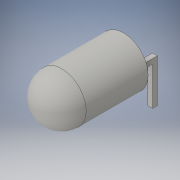
# Autodesk Inventor part: LED
Saved by Autodesk Inventor 2016 (Build 200138000, 138)
## iProperties
Created: 2017-05-28
Part Number: LED
Material: 一般
Document SubType Name: Modeling
Designer: kota
Density: 1 g/cm^3
Appearance: 既定
Author: kota
Autodesk Inventor part; units mm, degrees
ref_plane "YZ Plane" through (0, 0, 0) normal (1, 0, 0) x (0, 1, 0)
ref_plane "XZ Plane" through (0, 0, 0) normal (0, 1, 0) x (-1, 0, 0)
ref_plane "XY Plane" through (0, 0, 0) normal (0, 0, 1) x (1, 0, 0)
sketch "スケッチ1" plane through (0, 0, 0) normal (0, 1, 0) x (-1, 0, 0)
  line L0 (4.5, 2.55) -> (-4.5, 2.55) construction
  line L1 (-4.5, 2.55) -> (-4.5, -2.55) construction
  line L2 (-4.5, -2.55) -> (4.5, -2.55) construction
  line L3 (4.5, -2.55) -> (4.5, 2.55) construction
  line L4 (4.5, 2.55) -> (-4.5, -2.55) construction
  line L5 (-4.5, 2.55) -> (4.5, -2.55) construction
  line L6 (5.4458, 0) -> (-6.2593, 0)
  line L7 (4.5, 0) -> (-4.5, 0)
  arc A0 (4.5, 0) -> (1.95, 2.55) centre (1.95, 0) ccw
  line L8 (-4.5, 2.55) -> (-4.5, 0)
  line L9 (1.95, 2.55) -> (-4.5, 2.55)
  point P0 (0, 0)
  dimension "d0" = 9
  dimension "d1" = 5.1
  constraints: 20 end point, 3 midpoint, 2 collinear, 2 horizontal, 2 parallel, 2 point on circle, 2 point on line, 2 tangent, 1 centre point, 1 perpendicular, 2 other
  measures "d0" distance of L2.end L1.end
  measures "d1" distance of L0.end L1.end
revolve "回転1" add sketch "スケッチ1" angle 360 about axis through (-5.4458, 0, 0) along (1, 0, 0)
sketch "スケッチ2" plane through (4.5, 0, 0) normal (1, 0, 0) x (0, 0, -1)
  line L0 (-3.2936, 0) -> (3.5532, 0)
  line L1 (0, -3.9082) -> (0, 3.9846)
  line L2 (-1.52, 0.25) -> (-1.02, 0.25)
  line L3 (-1.02, 0.25) -> (-1.02, -0.25)
  line L4 (-1.02, -0.25) -> (-1.52, -0.25)
  line L5 (-1.52, -0.25) -> (-1.52, 0.25)
  line L6 (-1.52, 0.25) -> (-1.02, -0.25) construction
  line L7 (-1.02, 0.25) -> (-1.52, -0.25) construction
  line L8 (1.52, 0.25) -> (1.02, 0.25)
  line L9 (1.02, 0.25) -> (1.02, -0.25)
  line L10 (1.02, -0.25) -> (1.52, -0.25)
  line L11 (1.52, 0.25) -> (1.02, -0.25) construction
  line L12 (1.02, 0.25) -> (1.52, -0.25) construction
  line L13 (1.52, -0.25) -> (1.52, 0.25)
  point P0 (0, 0)
  point P1 (-1.27, 0)
  point P2 (-1.27, 0)
  point P3 (1.27, 0)
  point P4 (1.27, 0)
  dimension "d9" = 0.5
  dimension "d10" = 0.5
  dimension "d11" = 1.27
  constraints: 28 end point, 6 symmetric about line, 5 midpoint, 3 horizontal, 2 parallel, 1 perpendicular, 1 point on line, 1 vertical, 4 other
  measures "d9" distance of L3.end L4.end
  measures "d10" distance of L2.end L3.end
  measures "d11" distance of point (0, 0) point (-1.27, 0)
extrude "押し出し1" add sketch "スケッチ2" along normal blind 2
sketch "スケッチ3" plane through (4.5, -0.25, 1.02) normal (0, -1, 0) x (1, 0, 0)
  line L0 (1.5, 0) -> (2, 0)
  line L1 (2, 0) -> (2, 0.5)
  line L2 (2, 0.5) -> (1.5, 0.5)
  line L3 (1.5, 0.5) -> (1.5, 0)
  line L4 (1.5, 0) -> (2, 0.5) construction
  line L5 (2, 0) -> (1.5, 0.5) construction
  line L6 (1.5, -2.04) -> (2, -2.04)
  line L7 (2, -2.04) -> (2, -2.54)
  line L8 (2, -2.54) -> (1.5, -2.54)
  line L9 (1.5, -2.54) -> (1.5, -2.04)
  line L10 (1.5, -2.04) -> (2, -2.54) construction
  line L11 (2, -2.04) -> (1.5, -2.54) construction
  point P0 (-4.5, -1.02)
  point P1 (1.75, 0.25)
  point P2 (1.75, -2.29)
  dimension "d14" = 0.5
  dimension "d15" = 0.5
  dimension "d16" = 0.5
  dimension "d17" = 0.5
  constraints: 24 end point, 4 midpoint, 4 parallel, 2 coincident, 2 horizontal, 2 perpendicular
  measures "d14" distance of L2.end L1.end
  measures "d15" distance of L1.end L0.end
  measures "d16" distance of L7.end L8.end
  measures "d17" distance of L6.end L7.end
extrude "押し出し2" add sketch "スケッチ3" along normal blind 4
